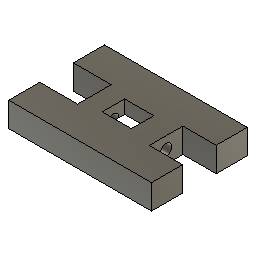
USAXS_flow cell holder v5 (Autodesk Fusion 360 design; units mm, degrees)
Autodesk Fusion 360 part; units mm, degrees
sketch "Sketch1" plane through (0, 0, 0) normal (0, 0, 1) x (1, 0, 0)
  line L0 (0, 0) -> (127.5, 0)
  line L1 (127.5, 0) -> (127.5, 85.5)
  line L2 (127.5, 85.5) -> (0, 85.5)
  line L3 (0, 85.5) -> (0, 0)
  dimension "d1" = 127.5
  dimension "d2" = 85.5
  constraint horizontal L0
  constraint vertical L1
  constraint horizontal L2
  constraint vertical L3
  constraint coincident L0.start L3.end
  measures "d1" distance of L0.start L0.end
  measures "d2" distance of L0.start L2.end
extrude "Extrude1" add sketch "Sketch1" along normal blind 22
sketch "Sketch2" plane through (0, 0, 22) normal (0, 0, 1) x (-1, 0, 0)
  line L0 (0, -85.5) -> (0, 0)
  line L1 (0, 0) -> (-127.5, 0)
  line L2 (-127.5, 0) -> (-127.5, -85.5)
  line L3 (-127.5, -85.5) -> (0, -85.5)
  line L4 (-76.75, -32.75) -> (-50.75, -32.75)
  line L5 (-50.75, -32.75) -> (-50.75, -52.75)
  line L6 (-50.75, -52.75) -> (-76.75, -52.75)
  line L7 (-76.75, -52.75) -> (-76.75, -32.75)
  line L8 (-76.75, -32.75) -> (-50.75, -52.75) construction
  line L9 (-50.75, -32.75) -> (-76.75, -52.75) construction
  point P0 (-63.75, -42.75)
  point P1 (-63.75, -42.75)
  dimension "d5" = 26
  dimension "d6" = 20
  constraint horizontal L4
  constraint perpendicular L4 L5
  constraint parallel L4 L6
  constraint parallel L5 L7
  constraint coincident L8 P1
  constraint coincident L9 P1
  constraint coincident P1 P0
  measures "d5" distance of L5.end L6.end
  measures "d6" distance of L4.end L5.end
extrude "Extrude2" cut sketch "Sketch2" against normal blind 25 contours L4 L5 L6 L7
sketch "Sketch3" plane through (0, 0, 22) normal (0, 0, 1) x (-1, 0, 0)
  line L0 (-50.75, -32.75) -> (-50.75, -52.75)
  line L1 (-50.75, -52.75) -> (-76.75, -52.75)
  line L2 (-76.75, -52.75) -> (-76.75, -32.75)
  line L3 (-76.75, -32.75) -> (-50.75, -32.75)
  line L4 (0, -85.5) -> (0, 0)
  line L5 (0, 0) -> (-127.5, 0)
  line L6 (-127.5, 0) -> (-127.5, -85.5)
  line L7 (-127.5, -85.5) -> (0, -85.5)
  line L8 (0, -27.75) -> (-33.75, -27.75)
  line L9 (-33.75, -27.75) -> (-33.75, -57.75)
  line L10 (-33.75, -57.75) -> (0, -57.75)
  line L11 (0, -57.75) -> (0, -27.75)
  point P0 (-33.75, -42.75)
  point P1 (0, -27.75)
  dimension "d9" = 33.75
  dimension "d10" = 30
  constraint coincident L4 P1
  constraint horizontal L8
  constraint vertical L9
  constraint horizontal L10
  constraint vertical L11
  constraint coincident P1 L8.start
  measures "d9" distance of P1 L8.end
  measures "d10" distance of P1 L10.end
extrude "Extrude3" cut sketch "Sketch3" against normal blind 300 contours L4 L8 L9 L10 L11
sketch "Sketch4" plane through (0, 0, 22) normal (0, 0, 1) x (-1, 0, 0)
  line L0 (-33.75, -27.75) -> (0, -27.75)
  line L1 (0, -27.75) -> (0, 0)
  line L2 (0, 0) -> (-127.5, 0)
  line L3 (-127.5, 0) -> (-127.5, -85.5)
  line L4 (-127.5, -85.5) -> (0, -85.5)
  line L5 (0, -85.5) -> (0, -57.75)
  line L6 (0, -57.75) -> (-33.75, -57.75)
  line L7 (-33.75, -57.75) -> (-33.75, -27.75)
  line L8 (-50.75, -32.75) -> (-50.75, -52.75)
  line L9 (-50.75, -52.75) -> (-76.75, -52.75)
  line L10 (-76.75, -52.75) -> (-76.75, -32.75)
  line L11 (-76.75, -32.75) -> (-50.75, -32.75)
  line L12 (-127.5, -27.75) -> (-97.75, -27.75)
  line L13 (-97.75, -27.75) -> (-97.75, -57.75)
  line L14 (-97.75, -57.75) -> (-127.5, -57.75)
  line L15 (-127.5, -57.75) -> (-127.5, -27.75)
  point P0 (-127.5, -27.75)
  dimension "d13" = 29.75
  dimension "d14" = 30
  constraint coincident L3 P0
  constraint horizontal L12
  constraint vertical L13
  constraint horizontal L14
  constraint vertical L15
  constraint coincident P0 L12.start
  measures "d13" distance of P0 L12.end
  measures "d14" distance of P0 L14.end
extrude "Extrude4" cut sketch "Sketch4" against normal blind 30 contours L3 L12 L13 L14 L15
sketch "Sketch5" plane through (97.75, 0, 0) normal (1, 0, 0) x (0, 1, 0)
  line L0 (27.75, 0) -> (57.75, 0)
  line L1 (57.75, 0) -> (57.75, 22)
  line L2 (57.75, 22) -> (27.75, 22)
  line L3 (27.75, 22) -> (27.75, 0)
  circle A0 centre (42.75, 11) radius 5.05
  point P0 (42.75, 11)
  dimension "d17" = 10.1
  constraint coincident P0 A0.centre
  measures "d17" diameter of A0
extrude "Extrude5" cut sketch "Sketch5" against normal blind 35 contours A0
sketch "Sketch6" plane through (33.75, 0, 0) normal (-1, 0, 0) x (0, -1, 0)
  line L0 (-57.75, 0) -> (-27.75, 0)
  line L1 (-27.75, 0) -> (-27.75, 22)
  line L2 (-27.75, 22) -> (-57.75, 22)
  line L3 (-57.75, 22) -> (-57.75, 0)
  circle A0 centre (-42.75, 11) radius 4.55
  point P0 (-42.75, 11)
  dimension "d20" = 9.1
  constraint coincident P0 A0.centre
  measures "d20" diameter of A0
extrude "Extrude6" cut sketch "Sketch6" against normal blind 25 contours A0
sketch "Sketch7" plane through (97.75, 0, 0) normal (1, 0, 0) x (0, 1, 0)
  circle A0 centre (42.75, 11) radius 5.05
  line L0 (27.75, 0) -> (57.75, 0)
  line L1 (57.75, 0) -> (57.75, 22)
  line L2 (57.75, 22) -> (27.75, 22)
  line L3 (27.75, 22) -> (27.75, 0)
  line L4 (32.5, 11.5) -> (42.5, 11.5)
  line L5 (42.5, 11.5) -> (42.5, 10.5)
  line L6 (42.5, 10.5) -> (32.5, 10.5)
  line L7 (32.5, 10.5) -> (32.5, 11.5)
  line L8 (32.5, 11.5) -> (42.5, 10.5) construction
  line L9 (42.5, 11.5) -> (32.5, 10.5) construction
  point P0 (37.5, 11)
  point P1 (37.5, 11)
  dimension "d23" = 10
  dimension "d24" = 1
  constraint horizontal L4
  constraint perpendicular L4 L5
  constraint parallel L4 L6
  constraint parallel L5 L7
  constraint coincident L8 P1
  constraint coincident L9 P1
  constraint coincident P1 P0
  measures "d23" distance of L5.end L6.end
  measures "d24" distance of L4.end L5.end
extrude "Extrude7" cut sketch "Sketch7" against normal blind 14 contours A0 L4 L6 L7
chamfer "Chamfer1" distance 10 angle 45 2 edges at (63.75, 52.75, 0) (63.75, 32.75, 0)
chamfer "Chamfer2" distance 10 angle 45 2 edges at (50.75, 42.75, 0) (76.75, 42.75, 0)
sketch "Sketch8" plane through (0, 0, 0) normal (0, 0, -1) x (1, 0, 0)
  line L0 (86.75, -62.75) -> (40.75, -62.75)
  line L1 (40.75, -62.75) -> (40.75, -22.75)
  line L2 (40.75, -22.75) -> (86.75, -22.75)
  line L3 (86.75, -22.75) -> (86.75, -62.75)
  line L4 (127.5, -57.75) -> (97.75, -57.75)
  line L5 (97.75, -57.75) -> (97.75, -27.75)
  line L6 (97.75, -27.75) -> (127.5, -27.75)
  line L7 (127.5, -27.75) -> (127.5, 0)
  line L8 (127.5, 0) -> (0, 0)
  line L9 (0, 0) -> (0, -27.75)
  line L10 (0, -27.75) -> (33.75, -27.75)
  line L11 (33.75, -27.75) -> (33.75, -57.75)
  line L12 (33.75, -57.75) -> (0, -57.75)
  line L13 (0, -57.75) -> (0, -85.5)
  line L14 (0, -85.5) -> (127.5, -85.5)
  line L15 (127.5, -85.5) -> (127.5, -57.75)
  point P0 (20, -65)
  point P1 (20, -20)
  constraint vertical P0 P1
hole "Hole1" at (20, 65, 0) at (20, 20, 0) direction (0, 0, 1) diameter 2.75 depth 11 tip angle 118
